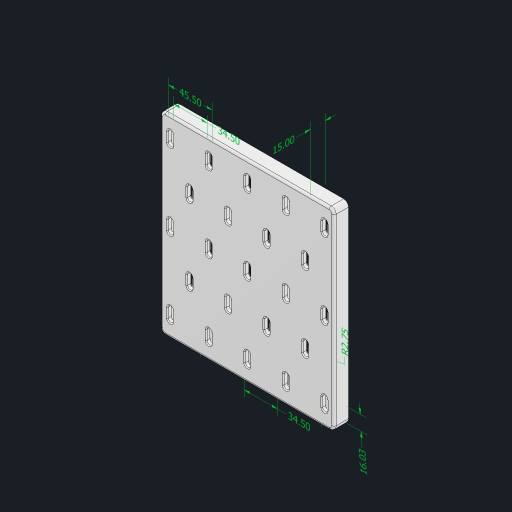
# Autodesk Inventor part: SKÅDIS Pegboard
Saved by Autodesk Inventor 2024 (Build 280153000, 153)
## iProperties
Created: 2024-02-06
Part Number: SKÅDIS Pegboard
Material: 일반
Document SubType Name: Modeling
Designer: KBU
Density: 1 g/cm^3
Appearance: 기본값
Author: KBU
Autodesk Inventor part; units mm, degrees
ref_plane "YZ Plane" through (0, 0, 0) normal (1, 0, 0) x (0, 1, 0)
ref_plane "XZ Plane" through (0, 0, 0) normal (0, 1, 0) x (-1, 0, 0)
ref_plane "XY Plane" through (0, 0, 0) normal (0, 0, 1) x (1, 0, 0)
sketch "스케치1" plane through (0, 0, 0) normal (0, 0, 1) x (1, 0, 0)
  line L0 (-110, -100) -> (110, -100)
  line L1 (110, -100) -> (110, 100)
  line L2 (110, 100) -> (-110, 100)
  line L3 (-110, 100) -> (-110, -100)
  line L4 (-110, -100) -> (110, 100) construction
  line L5 (110, -100) -> (-110, 100) construction
  line L6 (-100, 74) -> (-100, 84) construction
  line L7 (-102.75, 74) -> (-102.75, 84)
  line L8 (-97.25, 84) -> (-97.25, 74)
  arc A0 (-102.75, 74) -> (-97.25, 74) centre (-100, 74) ccw
  arc A1 (-97.25, 84) -> (-102.75, 84) centre (-100, 84) ccw
  line L9 (-62.75, 74) -> (-62.75, 84)
  line L10 (-60, 74) -> (-60, 84) construction
  line L11 (-57.25, 84) -> (-57.25, 74)
  arc A2 (-62.75, 74) -> (-57.25, 74) centre (-60, 74) ccw
  arc A3 (-57.25, 84) -> (-62.75, 84) centre (-60, 84) ccw
  line L12 (-22.75, 74) -> (-22.75, 84)
  line L13 (-20, 74) -> (-20, 84) construction
  line L14 (-17.25, 84) -> (-17.25, 74)
  arc A4 (-22.75, 74) -> (-17.25, 74) centre (-20, 74) ccw
  arc A5 (-17.25, 84) -> (-22.75, 84) centre (-20, 84) ccw
  line L15 (17.25, 74) -> (17.25, 84)
  line L16 (20, 74) -> (20, 84) construction
  line L17 (22.75, 84) -> (22.75, 74)
  arc A6 (17.25, 74) -> (22.75, 74) centre (20, 74) ccw
  arc A7 (22.75, 84) -> (17.25, 84) centre (20, 84) ccw
  line L18 (57.25, 74) -> (57.25, 84)
  line L19 (60, 74) -> (60, 84) construction
  line L20 (62.75, 84) -> (62.75, 74)
  arc A8 (57.25, 74) -> (62.75, 74) centre (60, 74) ccw
  arc A9 (62.75, 84) -> (57.25, 84) centre (60, 84) ccw
  line L21 (97.25, 74) -> (97.25, 84)
  line L22 (100, 74) -> (100, 84) construction
  line L23 (102.75, 84) -> (102.75, 74)
  arc A10 (97.25, 74) -> (102.75, 74) centre (100, 74) ccw
  arc A11 (102.75, 84) -> (97.25, 84) centre (100, 84) ccw
  line L24 (-80, 34.5) -> (-80, 44.5) construction
  line L25 (-77.25, 34.5) -> (-77.25, 44.5)
  line L26 (-82.75, 44.5) -> (-82.75, 34.5)
  arc A12 (-82.75, 34.5) -> (-77.25, 34.5) centre (-80, 34.5) ccw
  arc A13 (-77.25, 44.5) -> (-82.75, 44.5) centre (-80, 44.5) ccw
  arc A14 (-37.25, 44.5) -> (-42.75, 44.5) centre (-40, 44.5) ccw
  line L27 (-42.75, 44.5) -> (-42.75, 34.5)
  line L28 (-40, 34.5) -> (-40, 44.5) construction
  arc A15 (-42.75, 34.5) -> (-37.25, 34.5) centre (-40, 34.5) ccw
  line L29 (-37.25, 34.5) -> (-37.25, 44.5)
  arc A16 (2.75, 44.5) -> (-2.75, 44.5) centre (0, 44.5) ccw
  line L30 (-2.75, 44.5) -> (-2.75, 34.5)
  line L31 (0, 34.5) -> (0, 44.5) construction
  arc A17 (-2.75, 34.5) -> (2.75, 34.5) centre (0, 34.5) ccw
  line L32 (2.75, 34.5) -> (2.75, 44.5)
  arc A18 (42.75, 44.5) -> (37.25, 44.5) centre (40, 44.5) ccw
  line L33 (37.25, 44.5) -> (37.25, 34.5)
  line L34 (40, 34.5) -> (40, 44.5) construction
  arc A19 (37.25, 34.5) -> (42.75, 34.5) centre (40, 34.5) ccw
  line L35 (42.75, 34.5) -> (42.75, 44.5)
  arc A20 (82.75, 44.5) -> (77.25, 44.5) centre (80, 44.5) ccw
  line L36 (77.25, 44.5) -> (77.25, 34.5)
  line L37 (80, 34.5) -> (80, 44.5) construction
  arc A21 (77.25, 34.5) -> (82.75, 34.5) centre (80, 34.5) ccw
  line L38 (82.75, 34.5) -> (82.75, 44.5)
  line L39 (-100, -5) -> (-100, 5) construction
  line L40 (-102.75, -5) -> (-102.75, 5)
  arc A22 (-102.75, -5) -> (-97.25, -5) centre (-100, -5) ccw
  arc A23 (-97.25, 5) -> (-102.75, 5) centre (-100, 5) ccw
  line L41 (-97.25, 5) -> (-97.25, -5)
  line L42 (-62.75, -5) -> (-62.75, 5)
  line L43 (-60, -5) -> (-60, 5) construction
  arc A24 (-57.25, 5) -> (-62.75, 5) centre (-60, 5) ccw
  line L44 (-57.25, 5) -> (-57.25, -5)
  arc A25 (-62.75, -5) -> (-57.25, -5) centre (-60, -5) ccw
  line L45 (-22.75, -5) -> (-22.75, 5)
  line L46 (-20, -5) -> (-20, 5) construction
  line L47 (-17.25, 5) -> (-17.25, -5)
  arc A26 (-22.75, -5) -> (-17.25, -5) centre (-20, -5) ccw
  arc A27 (-17.25, 5) -> (-22.75, 5) centre (-20, 5) ccw
  line L48 (17.25, -5) -> (17.25, 5)
  line L49 (20, -5) -> (20, 5) construction
  arc A28 (17.25, -5) -> (22.75, -5) centre (20, -5) ccw
  line L50 (22.75, 5) -> (22.75, -5)
  arc A29 (22.75, 5) -> (17.25, 5) centre (20, 5) ccw
  line L51 (57.25, -5) -> (57.25, 5)
  line L52 (60, -5) -> (60, 5) construction
  line L53 (62.75, 5) -> (62.75, -5)
  arc A30 (57.25, -5) -> (62.75, -5) centre (60, -5) ccw
  arc A31 (62.75, 5) -> (57.25, 5) centre (60, 5) ccw
  line L54 (97.25, -5) -> (97.25, 5)
  line L55 (100, -5) -> (100, 5) construction
  arc A32 (97.25, -5) -> (102.75, -5) centre (100, -5) ccw
  line L56 (102.75, 5) -> (102.75, -5)
  arc A33 (102.75, 5) -> (97.25, 5) centre (100, 5) ccw
  line L57 (-100, -84) -> (-100, -74) construction
  line L58 (-102.75, -84) -> (-102.75, -74)
  arc A34 (-102.75, -84) -> (-97.25, -84) centre (-100, -84) ccw
  arc A35 (-97.25, -74) -> (-102.75, -74) centre (-100, -74) ccw
  line L59 (-97.25, -74) -> (-97.25, -84)
  line L60 (-62.75, -84) -> (-62.75, -74)
  line L61 (-60, -84) -> (-60, -74) construction
  arc A36 (-57.25, -74) -> (-62.75, -74) centre (-60, -74) ccw
  line L62 (-57.25, -74) -> (-57.25, -84)
  arc A37 (-62.75, -84) -> (-57.25, -84) centre (-60, -84) ccw
  line L63 (-22.75, -84) -> (-22.75, -74)
  line L64 (-20, -84) -> (-20, -74) construction
  line L65 (-17.25, -74) -> (-17.25, -84)
  arc A38 (-22.75, -84) -> (-17.25, -84) centre (-20, -84) ccw
  arc A39 (-17.25, -74) -> (-22.75, -74) centre (-20, -74) ccw
  line L66 (17.25, -84) -> (17.25, -74)
  line L67 (20, -84) -> (20, -74) construction
  arc A40 (17.25, -84) -> (22.75, -84) centre (20, -84) ccw
  line L68 (22.75, -74) -> (22.75, -84)
  arc A41 (22.75, -74) -> (17.25, -74) centre (20, -74) ccw
  line L69 (57.25, -84) -> (57.25, -74)
  line L70 (60, -84) -> (60, -74) construction
  line L71 (62.75, -74) -> (62.75, -84)
  arc A42 (57.25, -84) -> (62.75, -84) centre (60, -84) ccw
  arc A43 (62.75, -74) -> (57.25, -74) centre (60, -74) ccw
  line L72 (97.25, -84) -> (97.25, -74)
  line L73 (100, -84) -> (100, -74) construction
  arc A44 (97.25, -84) -> (102.75, -84) centre (100, -84) ccw
  line L74 (102.75, -74) -> (102.75, -84)
  arc A45 (102.75, -74) -> (97.25, -74) centre (100, -74) ccw
  line L75 (-80, -44.5) -> (-80, -34.5) construction
  line L76 (-77.25, -44.5) -> (-77.25, -34.5)
  arc A46 (-82.75, -44.5) -> (-77.25, -44.5) centre (-80, -44.5) ccw
  arc A47 (-77.25, -34.5) -> (-82.75, -34.5) centre (-80, -34.5) ccw
  line L77 (-82.75, -34.5) -> (-82.75, -44.5)
  arc A48 (2.75, -34.5) -> (-2.75, -34.5) centre (0, -34.5) ccw
  line L78 (2.75, -44.5) -> (2.75, -34.5)
  line L79 (0, -44.5) -> (0, -34.5) construction
  line L80 (-2.75, -34.5) -> (-2.75, -44.5)
  arc A49 (-2.75, -44.5) -> (2.75, -44.5) centre (0, -44.5) ccw
  arc A50 (42.75, -34.5) -> (37.25, -34.5) centre (40, -34.5) ccw
  line L81 (37.25, -34.5) -> (37.25, -44.5)
  line L82 (40, -44.5) -> (40, -34.5) construction
  line L83 (42.75, -44.5) -> (42.75, -34.5)
  arc A51 (37.25, -44.5) -> (42.75, -44.5) centre (40, -44.5) ccw
  arc A52 (82.75, -34.5) -> (77.25, -34.5) centre (80, -34.5) ccw
  line L84 (80, -44.5) -> (80, -34.5) construction
  line L85 (77.25, -34.5) -> (77.25, -44.5)
  arc A53 (77.25, -44.5) -> (82.75, -44.5) centre (80, -44.5) ccw
  line L86 (82.75, -44.5) -> (82.75, -34.5)
  arc A54 (-37.25, -34.5) -> (-42.75, -34.5) centre (-40, -34.5) ccw
  line L87 (-42.75, -34.5) -> (-42.75, -44.5)
  line L88 (-40, -44.5) -> (-40, -34.5) construction
  arc A55 (-42.75, -44.5) -> (-37.25, -44.5) centre (-40, -44.5) ccw
  line L89 (-37.25, -44.5) -> (-37.25, -34.5)
  line L90 (70, -100) -> (70, 100)
  point P0 (0, 0)
  point P1 (-100, 79)
  point P2 (-100, 71.25)
  point P3 (-100, 86.75)
  point P4 (-60, 79)
  point P5 (-60, 71.25)
  point P6 (-60, 86.75)
  point P7 (-20, 79)
  point P8 (-20, 71.25)
  point P9 (-20, 86.75)
  point P10 (20, 79)
  point P11 (20, 71.25)
  point P12 (20, 86.75)
  point P13 (60, 79)
  point P14 (60, 71.25)
  point P15 (60, 86.75)
  point P16 (100, 79)
  point P17 (100, 71.25)
  point P18 (100, 86.75)
  point P19 (100, 79)
  point P20 (-80, 39.5)
  point P21 (-80, 47.25)
  point P22 (-80, 31.75)
  point P23 (-40, 47.25)
  point P24 (-40, 39.5)
  point P25 (-40, 31.75)
  point P26 (0, 47.25)
  point P27 (0, 39.5)
  point P28 (0, 31.75)
  point P29 (40, 47.25)
  point P30 (40, 39.5)
  point P31 (40, 31.75)
  point P32 (80, 47.25)
  point P33 (80, 39.5)
  point P34 (80, 31.75)
  point P35 (-100, 0)
  point P36 (-100, -7.75)
  point P37 (-100, 7.75)
  point P38 (-60, 0)
  point P39 (-60, -7.75)
  point P40 (-60, 7.75)
  point P41 (-20, 0)
  point P42 (-20, -7.75)
  point P43 (-20, 7.75)
  point P44 (20, 0)
  point P45 (20, -7.75)
  point P46 (20, 7.75)
  point P47 (60, 0)
  point P48 (60, -7.75)
  point P49 (60, 7.75)
  point P50 (100, 0)
  point P51 (100, 0)
  point P52 (100, -7.75)
  point P53 (100, 7.75)
  point P54 (-100, -79)
  point P55 (-100, -86.75)
  point P56 (-100, -71.25)
  point P57 (-60, -79)
  point P58 (-60, -86.75)
  point P59 (-60, -71.25)
  point P60 (-20, -79)
  point P61 (-20, -86.75)
  point P62 (-20, -71.25)
  point P63 (20, -79)
  point P64 (20, -86.75)
  point P65 (20, -71.25)
  point P66 (60, -79)
  point P67 (60, -86.75)
  point P68 (60, -71.25)
  point P69 (100, -79)
  point P70 (100, -79)
  point P71 (100, -86.75)
  point P72 (100, -71.25)
  point P73 (-80, -39.5)
  point P74 (-80, -47.25)
  point P75 (-80, -31.75)
  point P76 (0, -31.75)
  point P77 (0, -39.5)
  point P78 (0, -47.25)
  point P79 (40, -31.75)
  point P80 (40, -39.5)
  point P81 (40, -47.25)
  point P82 (80, -31.75)
  point P83 (80, -39.5)
  point P84 (80, -47.25)
  point P85 (-40, -31.75)
  point P86 (-40, -39.5)
  point P87 (-40, -47.25)
  point P88 (100, -86.75)
  point P89 (-60, -86.75)
  point P90 (60, 79)
  dimension "d0" = 220
  dimension "d1" = 200
  dimension "d2" = 5.5
  dimension "d3" = 15.5
  dimension "d7" = 10
  dimension "d8" = 21
  dimension "d13" = 40
  dimension "d20" = 5.5
  dimension "d21" = 15.5
  dimension "d22" = 30
  dimension "d24" = 55
  dimension "d30" = 40
  dimension "d37" = 79
  dimension "d44" = 79
  dimension "d51" = 13.25
  dimension "d52" = 13.25
  dimension "d76" = 180
  dimension "d77" = 10
  constraints: 238 end point, 118 point on circle, 56 centre point, 8 tangent, 6 midpoint, 4 parallel, 4 vertical, 3 horizontal, 2 perpendicular, 2 point on line, 366 other
  measures "d0" distance of L1.end L2.end
  measures "d1" distance of L0.end L1.end
  measures "d2" distance between parallel lines of L8 L7
  measures "d3" distance of point (-100, 71.25) point (-100, 86.75)
  measures "d7" distance from line of point (-100, 79) L3
  measures "d8" distance from line of L2 point (-100, 79)
  measures "d13" distance of L7.start L9.start
  measures "d20" distance between parallel lines of L26 L25
  measures "d21" distance of point (-80, 47.25) point (-80, 31.75)
  measures "d22" distance from line of L3 point (-80, 39.5)
  measures "d24" vertical distance of point (-80, 31.75) point (-100, 86.75)
  measures "d30" distance of point (-80, 47.25) point (-40, 47.25)
  measures "d37" distance of point (-100, 79) point (-100, 0)
  measures "d44" distance of L24.start L75.start
  measures "d51" distance from line of L0 point (-60, -86.75)
  measures "d52" distance from line of L2 point (-100, 86.75)
  measures "d76" distance between parallel lines of L3 L90
  measures "d77" distance from line of L90 point (60, 79)
extrude "돌출1" add sketch "스케치1" along normal blind 5 contours L3 L2 L90 L0
sketch "스케치2" plane through (0, 0, 0) normal (0, 0, -1) x (-1, 0, 0)
  line L0 (-70, -100) -> (-70, 100) projected
  line L1 (110, -100) -> (-70, -100) projected
  line L2 (-70, 100) -> (110, 100)
  line L3 (110, 100) -> (110, -100)
  line L4 (110, -100) -> (-70, -100)
  line L5 (-70, -100) -> (-70, 100)
  line L6 (105, 95) -> (-65, 95)
  line L7 (-65, 95) -> (-65, -95)
  line L8 (-65, -95) -> (105, -95)
  line L9 (105, -95) -> (105, 95)
  line L10 (-12.5, 95) -> (-12.5, -95)
  line L11 (-17.25, -84) -> (-17.25, -74) projected
  line L12 (-7.5, -95) -> (-7.5, 95)
  line L13 (-2.75, -34.5) -> (-2.75, -44.5) projected
  line L14 (47.5, -95) -> (47.5, 95)
  line L15 (52.5, -95) -> (52.5, 95)
  line L16 (57.25, -74) -> (57.25, -84) projected
  line L17 (42.75, -44.5) -> (42.75, -34.5) projected
  point P0 (-2.75, -39.5)
  point P1 (57.25, -79)
  dimension "d79" = 5
  dimension "d80" = 4.75
  dimension "d81" = 4.75
  dimension "d82" = 5
  dimension "d83" = 4.75
  dimension "d84" = 4.75
  dimension "d85" = 5
  constraints: 24 end point, 6 point on line, 5 parallel, 5 perpendicular, 4 horizontal, 3 vertical, 2 midpoint, 8 other
  measures "d79" distance between parallel lines of L2 L6
  measures "d80" distance between parallel lines of L10 L11
  measures "d81" distance from line of L12 point (-2.75, -39.5)
  measures "d82" distance between parallel lines of L12 L10
  measures "d83" distance from line of point (57.25, -79) L15
  measures "d84" distance between parallel lines of L17 L14
  measures "d85" distance between parallel lines of L15 L14
extrude "돌출2" add sketch "스케치2" along normal blind 10 contours L0 L2 L3 L1 | L15 L8 L14 L6 | L12 L8 L10 L6
fillet "모깎기1" radius 5 4 edges at (-110, 100, -2.5) (70, -100, -2.5) (70, 100, -2.5) (-110, -100, -2.5)
fillet "모깎기2" radius 2.25 12 edges at (65, 95, -5) (12.5, 95, -5) (7.5, 95, -5) (-47.5, 95, -5) (-52.5, 95, -5) (-105, 95, -5) (-105, -95, -5) (-52.5, -95, -5) (-47.5, -95, -5) (7.5, -95, -5) (12.5, -95, -5) (65, -95, -5)
fillet "모깎기3" radius 1 184 edges at (-100, -86.75, 5) (-102.75, -79, 5) (-100, -71.25, 5) (-97.25, -79, 5) (-100, 71.25, 5) (-102.75, 79, 5) (-100, 86.75, 5) (-97.25, 79, 5) (-22.75, 79, 5) (-20, 86.75, 5) (-17.25, 79, 5) (-20, 71.25, 5) (-62.75, 79, 5) (-60, 86.75, 5) (-57.25, 79, 5) (-60, 71.25, 5) (17.25, 79, 5) (20, 86.75, 5) (22.75, 79, 5) (20, 71.25, 5) (57.25, 79, 5) (60, 86.75, 5) (62.75, 79, 5) (60, 71.25, 5) (37.25, 39.5, 5) (40, 47.25, 5) (42.75, 39.5, 5) (40, 31.75, 5) (-2.75, 39.5, 5) (0, 47.25, 5) (2.75, 39.5, 5) (0, 31.75, 5) (-40, 47.25, 5) (-37.25, 39.5, 5) (-40, 31.75, 5) (-42.75, 39.5, 5) (-82.75, 39.5, 5) (-80, 47.25, 5) (-77.25, 39.5, 5) (-80, 31.75, 5) (-100, -7.75, 5) (-102.75, 0, 5) (-100, 7.75, 5) (-97.25, 0, 5) (-60, -7.75, 5) (-62.75, 0, 5) (-60, 7.75, 5) (-57.25, 0, 5) (-20, 7.75, 5) (-17.25, 0, 5) (-20, -7.75, 5) (-22.75, 0, 5) (17.25, 0, 5) (20, 7.75, 5) (22.75, 0, 5) (20, -7.75, 5) (60, 7.75, 5) (62.75, 0, 5) (60, -7.75, 5) (57.25, 0, 5) (37.25, -39.5, 5) (40, -31.75, 5) (42.75, -39.5, 5) (40, -47.25, 5) (-2.75, -39.5, 5) (0, -31.75, 5) (2.75, -39.5, 5) (0, -47.25, 5) (-42.75, -39.5, 5) (-40, -31.75, 5) (-37.25, -39.5, 5) (-40, -47.25, 5) (-82.75, -39.5, 5) (-80, -31.75, 5) (-77.25, -39.5, 5) (-80, -47.25, 5) (-62.75, -79, 5) (-60, -71.25, 5) (-57.25, -79, 5) (-60, -86.75, 5) (-22.75, -79, 5) (-20, -71.25, 5) (-17.25, -79, 5) (-20, -86.75, 5) (17.25, -79, 5) (20, -71.25, 5) (22.75, -79, 5) (20, -86.75, 5) (57.25, -79, 5) (60, -71.25, 5) (62.75, -79, 5) (60, -86.75, 5) (57.25, 79, 0) (60, 86.75, 0) (62.75, 79, 0) (60, 71.25, 0) (20, 86.75, 0) (22.75, 79, 0) (20, 71.25, 0) (17.25, 79, 0) (-20, 71.25, 0) (-22.75, 79, 0) (-20, 86.75, 0) (-17.25, 79, 0) (-102.75, 79, 0) (-100, 86.75, 0) (-97.25, 79, 0) (-100, 71.25, 0) (-62.75, 79, 0) (-60, 86.75, 0) (-57.25, 79, 0) (-60, 71.25, 0) (-80, 31.75, 0) (-82.75, 39.5, 0) (-80, 47.25, 0) (-77.25, 39.5, 0) (-102.75, 0, 0) (-100, 7.75, 0) (-97.25, 0, 0) (-100, -7.75, 0) (-62.75, 0, 0) (-60, 7.75, 0) (-57.25, 0, 0) (-60, -7.75, 0) (-80, -31.75, 0) (-77.25, -39.5, 0) (-80, -47.25, 0) (-82.75, -39.5, 0) (-60, -71.25, 0) (-57.25, -79, 0) (-60, -86.75, 0) (-62.75, -79, 0) (-100, -86.75, 0) (-102.75, -79, 0) (-100, -71.25, 0) (-97.25, -79, 0) (-22.75, -79, 0) (-20, -71.25, 0) (-17.25, -79, 0) (-20, -86.75, 0) (20, -86.75, 0) (17.25, -79, 0) (20, -71.25, 0) (22.75, -79, 0) (40, -31.75, 0) (42.75, -39.5, 0) (40, -47.25, 0) (37.25, -39.5, 0) (0, -31.75, 0) (2.75, -39.5, 0) (0, -47.25, 0) (-2.75, -39.5, 0) (-40, -47.25, 0) (-42.75, -39.5, 0) (-40, -31.75, 0) (-37.25, -39.5, 0) (-20, 7.75, 0) (-17.25, 0, 0) (-20, -7.75, 0) (-22.75, 0, 0) (-40, 31.75, 0) (-42.75, 39.5, 0) (-40, 47.25, 0) (-37.25, 39.5, 0) (0, 31.75, 0) (-2.75, 39.5, 0) (0, 47.25, 0) (2.75, 39.5, 0) (40, 47.25, 0) (42.75, 39.5, 0) (40, 31.75, 0) (37.25, 39.5, 0) (22.75, 0, 0) (20, -7.75, 0) (17.25, 0, 0) (20, 7.75, 0) (60, 7.75, 0) (62.75, 0, 0) (60, -7.75, 0) (57.25, 0, 0) (60, -86.75, 0) (57.25, -79, 0) (60, -71.25, 0) (62.75, -79, 0)
fillet "모깎기4" radius 2.25 4 edges at (-20, -100, 5) (-20, 100, 5) (-108.5355, 98.5355, 5) (-110, 0, 5)
sketch "스케치3" plane through (0, 0, -10) normal (0, 0, -1) x (-1, 0, 0)
  line L0 (105, 92.75) -> (105, -92.75) projected
  line L1 (110, 95) -> (110, -95) projected
  line L2 (-70, -95) -> (110, -95)
  line L3 (110, -95) -> (110, -63)
  line L4 (110, -63) -> (-70, -63)
  line L5 (-70, -63) -> (-70, -95)
  arc A0 (96.25, -84) -> (103.75, -84) centre (100, -84) ccw projected
  arc A1 (103.75, -74) -> (96.25, -74) centre (100, -74) ccw projected
  point P0 (0, 0)
  point P1 (100, -87.75)
  point P2 (100, -70.25)
  dimension "d86" = 7.25
  dimension "d87" = 7.25
  constraints: 8 end point, 2 parallel, 2 point on circle, 1 horizontal, 1 perpendicular, 1 point on line
  measures "d86" distance from line of point (100, -87.75) L2
  measures "d87" distance from line of L4 point (100, -70.25)
extrude "돌출3" add sketch "스케치3" against normal blind 5
fillet "모깎기5" radius 2.25 6 edges at (-105, -63, -7.5) (-52.5, -63, -7.5) (-47.5, -63, -7.5) (7.5, -63, -7.5) (12.5, -63, -7.5) (65, -63, -7.5)
sketch "스케치4" plane through (0, 0, -10) normal (0, 0, -1) x (-1, 0, 0)
  line L0 (-65, -100) -> (105, -100) projected
  line L1 (-40, -84) -> (-40, -74) construction
  line L2 (-37.25, -84) -> (-37.25, -74)
  line L3 (-42.75, -74) -> (-42.75, -84)
  arc A0 (-42.75, -84) -> (-37.25, -84) centre (-40, -84) ccw
  arc A1 (-37.25, -74) -> (-42.75, -74) centre (-40, -74) ccw
  arc A2 (-43.75, -44.5) -> (-36.25, -44.5) centre (-40, -44.5) ccw projected
  arc A3 (2.75, -74) -> (-2.75, -74) centre (0, -74) ccw
  line L4 (-2.75, -74) -> (-2.75, -84)
  line L5 (0, -84) -> (0, -74) construction
  arc A4 (-2.75, -84) -> (2.75, -84) centre (0, -84) ccw
  line L6 (2.75, -84) -> (2.75, -74)
  arc A5 (42.75, -74) -> (37.25, -74) centre (40, -74) ccw
  line L7 (37.25, -74) -> (37.25, -84)
  line L8 (40, -84) -> (40, -74) construction
  arc A6 (37.25, -84) -> (42.75, -84) centre (40, -84) ccw
  line L9 (42.75, -84) -> (42.75, -74)
  arc A7 (82.75, -74) -> (77.25, -74) centre (80, -74) ccw
  line L10 (77.25, -74) -> (77.25, -84)
  line L11 (80, -84) -> (80, -74) construction
  arc A8 (77.25, -84) -> (82.75, -84) centre (80, -84) ccw
  line L12 (82.75, -84) -> (82.75, -74)
  point P0 (0, 0)
  point P1 (-40, -79)
  point P2 (-40, -71.25)
  point P3 (-40, -86.75)
  point P4 (-40, -48.25)
  point P5 (0, -71.25)
  point P6 (0, -79)
  point P7 (0, -86.75)
  point P8 (40, -71.25)
  point P9 (40, -79)
  point P10 (40, -86.75)
  point P11 (80, -71.25)
  point P12 (80, -79)
  point P13 (80, -86.75)
  dimension "d91" = 5.5
  dimension "d92" = 15.5
  dimension "d93" = 13.25
  dimension "d96" = 40
  constraints: 32 end point, 19 point on circle, 8 centre point, 4 tangent, 1 horizontal, 1 midpoint, 1 parallel, 1 vertical, 1 vertical alignment, 42 other
  measures "d91" distance between parallel lines of L2 L3
  measures "d92" distance of point (-40, -71.25) point (-40, -86.75)
  measures "d93" distance from line of L0 point (-40, -86.75)
  measures "d96" distance of point (-40, -71.25) point (0, -71.25)
extrude "돌출6" cut sketch "스케치4" against normal up to surface (5 mm away)
fillet "모깎기10" radius 1 32 edges at (40, -86.75, -5) (37.25, -79, -5) (40, -71.25, -5) (42.75, -79, -5) (40, -71.25, -10) (37.25, -79, -10) (40, -86.75, -10) (42.75, -79, -10) (0, -86.75, -10) (2.75, -79, -10) (0, -71.25, -10) (-2.75, -79, -10) (0, -86.75, -5) (-2.75, -79, -5) (0, -71.25, -5) (2.75, -79, -5) (-40, -86.75, -5) (-42.75, -79, -5) (-40, -71.25, -5) (-37.25, -79, -5) (-40, -71.25, -10) (-42.75, -79, -10) (-40, -86.75, -10) (-37.25, -79, -10) (-80, -86.75, -5) (-82.75, -79, -5) (-80, -71.25, -5) (-77.25, -79, -5) (-80, -71.25, -10) (-82.75, -79, -10) (-80, -86.75, -10) (-77.25, -79, -10)
equation "\"d20\" = d2"
equation "\"d21\" = d3"
equation "\"d81\" = d80"
equation "\"d83\" = d80"
equation "\"d84\" = d80"
